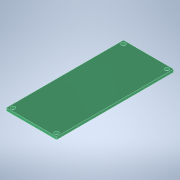
# Autodesk Inventor part: Lochrasterplatine
Saved by Autodesk Inventor 2021 (Build 250183000, 183)
## iProperties
Created: 2021-05-05
Part Number: Lochrasterplatine
Material: Generisch
Document SubType Name: Modeling
Designer: Maxim
Density: 1 g/cm^3
Appearance: Vorgabe
Author: Maxim
Autodesk Inventor part; units mm, degrees
ref_plane "YZ Plane" through (0, 0, 0) normal (1, 0, 0) x (0, 1, 0)
ref_plane "XZ Plane" through (0, 0, 0) normal (0, 1, 0) x (-1, 0, 0)
ref_plane "XY Plane" through (0, 0, 0) normal (0, 0, 1) x (1, 0, 0)
sketch "Skizze1" plane through (0, 0, 0) normal (0, 1, 0) x (-1, 0, 0)
  line L0 (-15, 35) -> (15, 35)
  line L1 (15, 35) -> (15, -35)
  line L2 (15, -35) -> (-15, -35)
  line L3 (-15, -35) -> (-15, 35)
  line L4 (-15, 35) -> (15, -35) construction
  line L5 (15, 35) -> (-15, -35) construction
  point P0 (0, 0)
  dimension "d0" = 70
  dimension "d1" = 30
  constraints: 12 end point, 2 midpoint, 2 parallel, 1 horizontal, 1 perpendicular
  measures "d0" distance of L0.end L1.end
  measures "d1" distance of L1.end L2.end
extrude "Extrusion1" add sketch "Skizze1" along normal blind 1.6
sketch "Skizze2" plane through (0, 0, 0) normal (0, 1, 0) x (-1, 0, 0)
  circle A0 centre (13, 33) radius 1.25
  line L0 (0, -40.6) -> (0, 40.6) projected
  line L1 (-26.6, 0) -> (26.6, 0) projected
  circle A1 centre (-13, 33) radius 1.25
  circle A2 centre (13, -33) radius 1.25
  circle A3 centre (-13, -33) radius 1.25
  point P0 (0, 0)
  dimension "d4" = 13
  dimension "d5" = 33
  dimension "d6" = 2.5
  dimension "d7" = 33
  dimension "d8" = 13
  dimension "d9" = 33
  dimension "d10" = 33
  dimension "d11" = 13
  dimension "d12" = 13
  dimension "d13" = 2.5
  dimension "d14" = 2.5
  dimension "d15" = 2.5
  constraints: 4 centre point
  measures "d4" distance from line of L0 A0.centre
  measures "d5" distance from line of L1 A0.centre
  measures "d6" diameter of A0
  measures "d7" distance from line of L1 A1.centre
  measures "d8" distance from line of L0 A1.centre
  measures "d9" distance from line of L1 A3.centre
  measures "d10" distance from line of L1 A2.centre
  measures "d11" distance from line of L0 A2.centre
  measures "d12" distance from line of L0 A3.centre
  measures "d13" diameter of A2
  measures "d14" diameter of A3
  measures "d15" diameter of A1
extrude "Extrusion2" add sketch "Skizze2" along normal blind 10 separate body
combine bodies "Kombinieren1" operation type subtract main body 1 bodies to subtract 2
